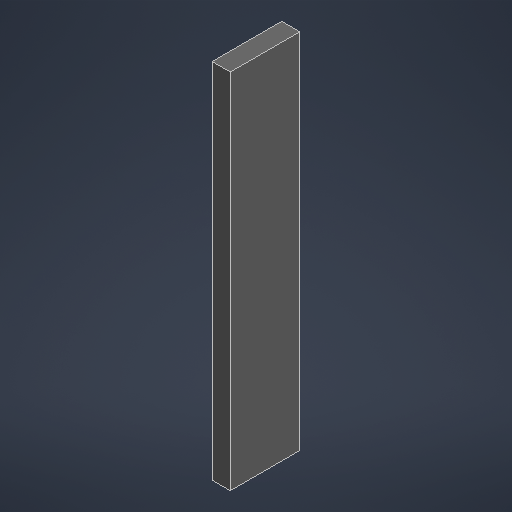
# Autodesk Inventor part: P_board
Saved by Autodesk Inventor 2026.2 (Build 302298000, 298)
## iProperties
Created: 2026-02-21
Part Number: P_board
Material: Generisch
Document SubType Name: Modeling
Designer: FAL
Density: 1 g/cm^3
Appearance: Vorgabe
Author: FAL
Autodesk Inventor part; units mm, degrees
ref_plane "YZ Plane" through (0, 0, 0) normal (1, 0, 0) x (0, 1, 0)
ref_plane "XZ Plane" through (0, 0, 0) normal (0, 1, 0) x (-1, 0, 0)
ref_plane "XY Plane" through (0, 0, 0) normal (0, 0, 1) x (1, 0, 0)
sketch "Skizze1" plane through (0, 0, 0) normal (1, 0, 0) x (0, 1, 0)
  line L0 (2.4, -12.5) -> (-2.4, -12.5)
  line L1 (-2.4, -12.5) -> (-2.4, 12.5)
  line L2 (-2.4, 12.5) -> (2.4, 12.5)
  line L3 (2.4, 12.5) -> (2.4, -12.5)
  line L4 (2.4, -12.5) -> (-2.4, 12.5) construction
  line L5 (-2.4, -12.5) -> (2.4, 12.5) construction
  point P0 (0, 0)
  dimension "d0" = 4.8
  dimension "d1" = 25
  constraints: 12 end point, 2 midpoint, 2 parallel, 1 horizontal, 1 perpendicular
  measures "d0" distance between parallel lines of L1 L3
  measures "d1" distance between parallel lines of L0 L2
extrude "Extrusion1" add sketch "Skizze1" along normal blind 1.25
